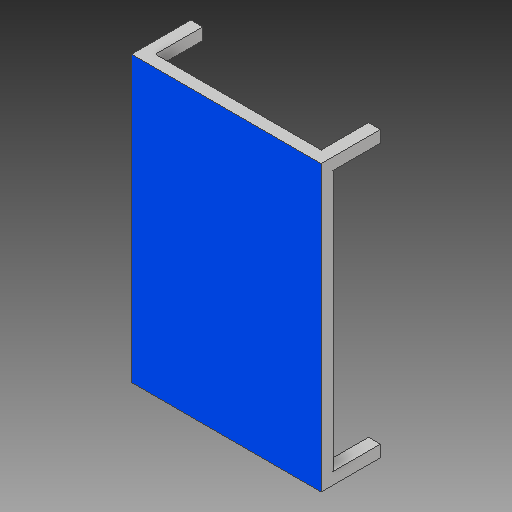
# Autodesk Inventor part: base_table
Saved by Autodesk Inventor 2018 (Build 220112000, 112)
## iProperties
Created: 2017-11-07
Part Number: base_table
Material: Generic
Document SubType Name: Modeling
Designer: kcmat
Density: 1 g/cm^3
Appearance: Default
Author: kcmat
Autodesk Inventor part; units mm, degrees
ref_plane "YZ Plane" through (0, 0, 0) normal (1, 0, 0) x (0, 1, 0)
ref_plane "XZ Plane" through (0, 0, 0) normal (0, 1, 0) x (-1, 0, 0)
ref_plane "XY Plane" through (0, 0, 0) normal (0, 0, 1) x (1, 0, 0)
sketch "Sketch1" plane through (0, 0, 0) normal (0, 0, 1) x (1, 0, 0)
  ellipse E0 centre (87.4656, 123.4744) end of major axis (87.4656, -181.3256) minor radius 228.6 projected
  line L0 (189.0656, 234.7689) -> (176.3656, 234.7689)
  line L1 (176.3656, 234.7689) -> (176.3656, 222.0689)
  line L2 (176.3656, 222.0689) -> (189.0656, 222.0689)
  line L3 (189.0656, 222.0689) -> (189.0656, 234.7689)
  line L4 (-14.1344, 234.7689) -> (-1.4344, 234.7689)
  line L5 (-1.4344, 234.7689) -> (-1.4344, 222.0689)
  line L6 (-1.4344, 222.0689) -> (-14.1344, 222.0689)
  line L7 (-14.1344, 222.0689) -> (-14.1344, 234.7689)
  line L8 (189.0656, -70.0311) -> (176.3656, -70.0311)
  line L9 (176.3656, -70.0311) -> (176.3656, -57.3311)
  line L10 (176.3656, -57.3311) -> (189.0656, -57.3311)
  line L11 (189.0656, -57.3311) -> (189.0656, -70.0311)
  line L12 (-14.1344, -70.0311) -> (-1.4344, -70.0311)
  line L13 (-1.4344, -70.0311) -> (-1.4344, -57.3311)
  line L14 (-1.4344, -57.3311) -> (-14.1344, -57.3311)
  line L15 (-14.1344, -57.3311) -> (-14.1344, -70.0311)
  line L16 (75.0457, -66.5884) -> (75.0457, -5.6676) projected
  line L17 (75.0457, -5.6676) -> (100.4457, -5.6676) projected
  line L18 (100.4457, -5.6676) -> (100.4457, -66.5884) projected
  line L19 (100.4457, -66.5884) -> (75.0457, -66.5884) projected
  circle A0 centre (87.4656, 239.7517) radius 30.4 projected
  point P0 (0, 0)
  dimension "d2" = 203.2
  dimension "d3" = 12.7
  dimension "d4" = 12.7
  dimension "d5" = 12.7
  dimension "d6" = 12.7
  dimension "d7" = 12.7
  constraints: 32 end point, 8 parallel, 4 horizontal, 4 perpendicular, 3 point on line, 1 other
  measures "d2" distance of L4.start L0.start
  measures "d3" distance of L2.end L1.end
  measures "d4" distance of L1.end L0.end
  measures "d5" distance of L5.end L6.end
  measures "d6" distance of L4.end L5.end
  measures "d7" distance of L8.end L9.end
extrude "Extrusion1" add sketch "Sketch1" along normal blind 50.8 contours L3 L2 L1 L0 | L4 L5 L6 L7 | L8 L9 L10 L11 | L15 L14 L13 L12
sketch "Sketch2" plane through (0, 0, 50.8) normal (0, 0, 1) x (1, 0, 0)
  line L0 (189.0656, 222.0689) -> (189.0656, 234.7689) projected
  line L1 (-14.1344, -70.0311) -> (-1.4344, -70.0311) projected
  line L2 (189.0656, 234.7689) -> (-14.1344, 234.7689)
  line L3 (-14.1344, 234.7689) -> (-14.1344, -70.0311)
  line L4 (-14.1344, -70.0311) -> (189.0656, -70.0311)
  line L5 (189.0656, -70.0311) -> (189.0656, 234.7689)
  point P0 (0, 0)
  constraints: 8 end point, 2 parallel, 1 horizontal, 1 perpendicular
extrude "Extrusion2" add sketch "Sketch2" along normal blind 12.7
body "Solid1"
